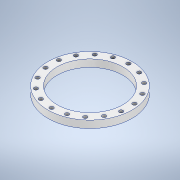
# Autodesk Inventor part: Injector Plate Retainer Ring
Saved by Autodesk Inventor 2021 (Build 250183000, 183)
## iProperties
Created: 2021-04-27
Part Number: Injector Plate Retainer Ring
Material: Aluminum 6061
Document SubType Name: Modeling
Designer: alexc
Mass: 151.621 g
Surface Area: 238.298 cm^2
Volume: 56.1559 cm^3
Density: 2.7 g/cm^3
Appearance: Aluminum - Flat
Author: alexc
Autodesk Inventor part; units mm, degrees
ref_plane "YZ Plane" through (0, 0, 0) normal (1, 0, 0) x (0, 1, 0)
ref_plane "XZ Plane" through (0, 0, 0) normal (0, 1, 0) x (-1, 0, 0)
sketch "Sketch1" plane through (0, 0, 0) normal (0, 1, 0) x (-1, 0, 0)
  circle A0 centre (0, 0) radius 57.15
  circle A1 centre (0, 0) radius 73.025
  dimension "d0" = 114.3
  dimension "d25" = 146.05
  constraints: 3 coincident, 2 centre point
  measures "d0" diameter of A0
  measures "d25" diameter of A1
extrude "Extrusion1" add sketch "Sketch1" along normal blind 12.7
sketch "Sketch4" plane through (0, 12.7, 0) normal (0, 1, 0) x (1, 0, 0)
  line L0 (0, 0) -> (0, -66.675) construction
  line L1 (0, 0) -> (0, -57.15) construction
  circle A0 centre (0, 0) radius 57.15 projected
  dimension "d14" = 66.675
  dimension "d33" = 0
  constraints: 4 end point, 1 vertical, 1 vertical alignment, 1 other
  measures "d14" distance of L0.end L0.start
  measures "d33" distance between parallel lines of L1 L0
hole "Hole2" at (0, 12.7, 66.675) direction (0, -1, 0) diameter 6.7564 end through all clearance for "Socket Head Cap Screw" size "1/4" standard "Ansi Unified Screw Threads"
pattern_circular "Circular Pattern2" count 18 over 360 about axis through (0, 0, 0) along (0, 1, 0) of "Hole2"
ref_plane "Work Plane1" through (0, 0, -69.85) normal (0, 0, 1) x (1, 0, 0)
body "Solid1"
